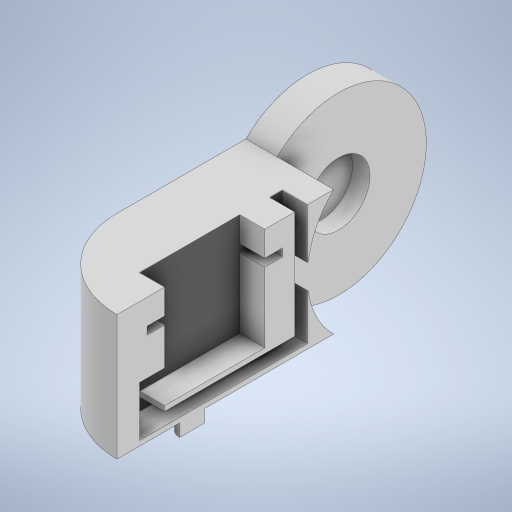
# Autodesk Inventor part: wirst 2 right
Saved by Autodesk Inventor 2023 (Build 270158000, 158)
## iProperties
Created: 2024-06-28
Part Number: wirst 2 right
Material: Generic
Document SubType Name: Modeling
Designer: Swoby
Density: 1 g/cm^3
Appearance: Default
Author: Swoby
Autodesk Inventor part; units mm, degrees
ref_plane "YZ Plane" through (0, 0, 0) normal (1, 0, 0) x (0, 1, 0)
ref_plane "XZ Plane" through (0, 0, 0) normal (0, 1, 0) x (-1, 0, 0)
ref_plane "XY Plane" through (0, 0, 0) normal (0, 0, 1) x (1, 0, 0)
sketch "Sketch1" plane through (0, 0, 0) normal (0, 1, 0) x (-1, 0, 0)
  arc A0 (35, -5) -> (0, 30) centre (0, -5) ccw
  line L0 (34.641, 0) -> (0, 0)
  line L1 (-35, -5) -> (-35, -100) construction
  line L2 (-35, -100) -> (0, -100) construction
  line L3 (35, -100) -> (35, -5)
  line L4 (0, -100) -> (0, 30)
  arc A1 (0, 30) -> (-35, -5) centre (0, -5) ccw construction
  line L5 (0, -5) -> (-35, -5) construction
  line L6 (0, -100) -> (35, -100)
  dimension "d0" = 70
  dimension "d1" = 130
  dimension "d32" = 30
  dimension "d33" = 35
  dimension "d34" = 5
  constraints: 14 end point, 5 parallel, 5 point on circle, 2 centre point, 2 horizontal, 2 perpendicular, 2 point on line, 1 vertical
  measures "d0" diameter of A0
  measures "d1" distance from line of L2 L4.end
  measures "d32" distance of point (0, 0) L4.end
  measures "d33" distance of L2.end L3.start
  measures "d34" vertical distance of point (0, 0) L3.end
extrude "Extrusion1" add sketch "Sketch1" along normal blind 50
sketch "Sketch2" plane through (0, 0, 30) normal (1, 0, 0) x (0, 0, -1)
  line L0 (19, 49) -> (27.5, 49)
  line L1 (59, 49) -> (59, 40)
  line L2 (59, 9) -> (19, 9)
  line L3 (19, 9) -> (19, 14)
  line L4 (19, 40) -> (12, 40)
  line L5 (12, 40) -> (12, 37)
  line L6 (12, 37) -> (19, 37)
  line L7 (19, 37) -> (19, 40) construction
  line L8 (19, 17) -> (14, 17)
  line L9 (14, 17) -> (14, 14)
  line L10 (14, 14) -> (19, 14)
  line L11 (19, 14) -> (19, 17) construction
  line L12 (59, 40) -> (66, 40)
  line L13 (66, 40) -> (66, 37)
  line L14 (66, 37) -> (59, 37)
  line L15 (59, 37) -> (59, 40) construction
  line L16 (27.5, 49) -> (32.5, 49) construction
  line L17 (32.5, 49) -> (32.5, 54)
  line L18 (32.5, 54) -> (27.5, 54)
  line L19 (27.5, 54) -> (27.5, 49)
  line L20 (0, 50) -> (130, 50) projected
  line L21 (19, 40) -> (19, 49)
  line L22 (19, 37) -> (19, 40) construction
  line L23 (19, 17) -> (19, 37)
  line L24 (19, 14) -> (19, 17) construction
  line L25 (59, 40) -> (59, 37) construction
  line L26 (59, 37) -> (59, 9)
  line L27 (27.5, 49) -> (32.5, 49) construction
  line L28 (32.5, 49) -> (59, 49)
  line L29 (9, 22) -> (19, 22)
  line L30 (19, 22) -> (19, 7)
  line L31 (19, 2) -> (9, 2)
  line L32 (9, 2) -> (9, 22)
  line L33 (19, 2) -> (76, 2)
  line L34 (19, 49) -> (19, 50)
  line L35 (59, 49) -> (59, 50)
  line L36 (71, 7) -> (71, 50)
  line L37 (71, 50) -> (76, 50)
  line L38 (76, 50) -> (76, 2)
  line L39 (71, 7) -> (19, 7)
  line L40 (0, 0) -> (0, 50) projected
  line L41 (30, 54) -> (30, 14.5)
  point P0 (66, 38.5)
  point P1 (19, 9)
  point P2 (32.5, 50)
  point P3 (27.5, 50)
  point P4 (19, 9)
  dimension "d5" = 3
  dimension "d6" = 3
  dimension "d7" = 5
  dimension "d8" = 40
  dimension "d9" = 5
  dimension "d10" = 5
  dimension "d11" = 36
  dimension "d12" = 40
  dimension "d13" = 7
  dimension "d14" = 5
  dimension "d15" = 7
  dimension "d16" = 9
  dimension "d18" = 1
  dimension "d20" = 10
  dimension "d21" = 5
  dimension "d22" = 20
  dimension "d26" = 5
  dimension "d27" = 5
  dimension "d28" = 57
  dimension "d29" = 48
  dimension "d30" = 5
  dimension "d36" = 30
  constraints: 80 end point, 31 parallel, 15 perpendicular, 9 horizontal, 2 midpoint, 2 point on line, 2 vertical, 1 collinear, 4 other
  measures "d5" distance between parallel lines of L6 L4
  measures "d6" distance of L8.end L9.end
  measures "d7" distance between parallel lines of L2 L10
  measures "d8" distance of L1.start L2.start
  measures "d9" distance of L17.end L18.end
  measures "d10" distance of L16.end L17.end
  measures "d11" horizontal distance of point (66, 38.5) L41.start
  measures "d12" distance of L0.start L1.start
  measures "d13" distance of L4.start L4.end
  measures "d14" distance of L8.start L8.end
  measures "d15" distance of L1.end L12.end
  measures "d16" distance between parallel lines of L0 L12
  measures "d20" distance of L29.start L29.end
  measures "d21" distance from line of L29 L8.end
  measures "d22" distance of L31.end L29.start
  measures "d26" distance between parallel lines of L38 L36
  measures "d27" distance between parallel lines of L33 L39
  measures "d28" distance of L33.end L31.start
  measures "d29" distance of L37.end L33.end
  measures "d30" distance from line of point (66, 38.5) L36
  measures "d36" distance between parallel lines of L40 L41
extrude "Extrusion2" cut sketch "Sketch2" against normal blind 10 contours L34 L20 L19 L0 | L0 L19 L20 L17 L28 L1 L12 L13 L14 L26 L2 L3 L30 L23 L6 L5 L4 L21 | L20 L35 L28 L17 | L23 L8 L9 L10 L3 L30 L39 L36 L20 L38 L33 L31 L32 L29 | L30 L10 L9 L8
sketch "Sketch3" plane through (-35, 0, -100) normal (-1, 0, 0) x (0, 0, 1)
  circle A0 centre (19, 25) radius 35
  line L0 (130, 0) -> (130, 50) projected
  line L1 (54, 50) -> (54, 2) projected
  line L2 (19, 25) -> (130, 25)
  point P0 (100, 0)
  dimension "d37" = 70
  constraints: 2 end point, 1 centre point, 1 midpoint, 1 perpendicular, 1 tangent
  measures "d37" diameter of A0
extrude "Extrusion3" add sketch "Sketch3" against normal up to surface (35 mm away)
sketch "Sketch4" plane through (0, 0, 0) normal (0, -1, 0) x (1, 0, 0)
  arc A0 (0, 5) -> (0, -5) centre (0, 0) ccw
  line L0 (0, 5) -> (0, -5)
  line L1 (0, -46) -> (0, 21) projected
  dimension "d41" = 10
  constraints: 2 end point, 2 point on circle, 2 point on line, 1 centre point, 1 coincident
  measures "d41" diameter of A0
extrude "Extrusion4" add sketch "Sketch4" along normal blind 5
sketch "Sketch5" plane through (0, 0, 30) normal (1, 0, 0) x (0, 0, -1)
  arc A0 (86.5051, 0) -> (86.5051, 50) centre (111, 25) ccw projected
  circle A1 centre (111, 25) radius 35
  line L0 (76, 30) -> (111, 30)
  line L1 (111, 30) -> (111, 20)
  line L2 (111, 20) -> (76, 20)
  line L3 (76, 20) -> (76, 30)
  line L4 (76, 50) -> (76, 2) projected
  point P0 (30, 0)
  point P1 (86.5051, 0)
  point P2 (76, 25)
  point P3 (76.359, 20)
  point P4 (76.359, 30)
  dimension "d46" = 10
  constraints: 8 end point, 2 midpoint, 2 parallel, 2 point on circle, 1 centre point, 1 coincident, 1 horizontal, 1 perpendicular, 1 point on line
  measures "d46" distance of L0.end L1.end
extrude "Extrusion5" cut sketch "Sketch5" against normal blind 22.5
sketch "Sketch6" plane through (-22.5, 0, 30) normal (1, 0, 0) x (0, 0, -1)
  arc A0 (86.5051, 0) -> (86.5051, 50) centre (111, 25) ccw projected
  circle A1 centre (111, 25) radius 12.5
  point P0 (30, 0)
  dimension "d47" = 25
  constraints: 1 centre point, 1 coincident
  measures "d47" diameter of A1
extrude "Extrusion6" cut sketch "Sketch6" against normal blind 7
equation "\"d33\" = 0.5 * d0"
equation "\"d34\" = 0.5 * d0 - d32"
body "Solid1"
